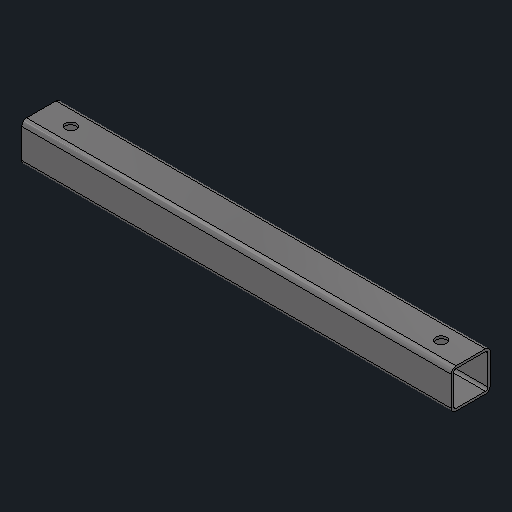
# Autodesk Inventor part: Model-4_Base Tube-1
Saved by Autodesk Inventor 2025.1 (Build 291241000, 241)
## iProperties
RuleStatus: InUse
Created: 2026-02-13
Part Number: Model-4_Base Tube-1
User Status: Released
Material: SS304
Description: Model-1 Base Tube-1
Document SubType Name: Modeling
Designer: Desktop -24
Density: 7.99949 g/cm^3
Appearance: Semi-Polished(1)
Mass: 20583.6 g
Surface Area: 8150.6 cm^2
Volume: 2573.11 cm^3
AfterDocNew0: Mat. Selection
encoded128: ÌStandard Î
encoded39: *STANDARD*
Family: SS304
Author: Desktop -24
Revision Number: 0
Autodesk Inventor part; units mm, degrees
ref_plane "YZ Plane" through (0, 0, 0) normal (1, 0, 0) x (0, 1, 0)
ref_plane "XZ Plane" through (0, 0, 0) normal (0, 1, 0) x (-1, 0, 0)
ref_plane "XY Plane" through (0, 0, 0) normal (0, 0, 1) x (1, 0, 0)
sketch "Sketch5" plane through (0, 0, 0) normal (1, 0, 0) x (0, 1, 0)
  line L0 (-38.1, 50.8) -> (38.1, 50.8)
  line L1 (50.8, 38.1) -> (50.8, -38.1)
  line L2 (38.1, -50.8) -> (-38.1, -50.8)
  line L3 (-50.8, -38.1) -> (-50.8, 38.1)
  line L4 (-50.8, 50.8) -> (50.8, -50.8) construction
  line L5 (50.8, 50.8) -> (-50.8, -50.8) construction
  arc A0 (50.8, 38.1) -> (38.1, 50.8) centre (38.1, 38.1) ccw
  arc A1 (38.1, -50.8) -> (50.8, -38.1) centre (38.1, -38.1) ccw
  arc A2 (-50.8, -38.1) -> (-38.1, -50.8) centre (-38.1, -38.1) ccw
  arc A3 (-38.1, 50.8) -> (-50.8, 38.1) centre (-38.1, 38.1) ccw
  line L6 (44.45, -38.1) -> (44.45, 38.1)
  arc A4 (44.45, 38.1) -> (38.1, 44.45) centre (38.1, 38.1) ccw
  line L7 (38.1, 44.45) -> (-38.1, 44.45)
  arc A5 (-38.1, 44.45) -> (-44.45, 38.1) centre (-38.1, 38.1) ccw
  line L8 (-44.45, 38.1) -> (-44.45, -38.1)
  arc A6 (-44.45, -38.1) -> (-38.1, -44.45) centre (-38.1, -38.1) ccw
  line L9 (-38.1, -44.45) -> (38.1, -44.45)
  arc A7 (38.1, -44.45) -> (44.45, -38.1) centre (38.1, -38.1) ccw
  point P0 (0, 0)
  dimension "d6" = 101.6
  dimension "d7" = 101.6
  dimension "d8" = 12.7
  dimension "d9" = 6.35
  constraints: 20 end point, 16 point on circle, 8 centre point, 8 point on line, 8 tangent, 4 parallel, 3 equal radius, 2 midpoint, 2 perpendicular, 1 horizontal, 7 other
  measures "d6" distance of L5.start L4.end
  measures "d7" distance of L4.end L5.end
  measures "d8" radius of A0
  measures "d9" distance between parallel lines of L1 L6
extrude "Extrusion4" add sketch "Sketch5" along normal mid plane 1111.25
sketch "Sketch9" plane through (-555.625, 50.8, 38.1) normal (0, 1, 0) x (1, 0, 0)
  line L0 (0, 38.1) -> (1111.25, 38.1) construction
  line L1 (1111.25, 0) -> (1111.25, 76.2) projected
  circle A0 centre (76.2, 38.1) radius 14.2875
  line L2 (0, 0) -> (0, 76.2) projected
  circle A1 centre (1035.05, 38.1) radius 14.2875
  point P0 (555.625, 38.1)
  dimension "d30" = 28.575
  dimension "d31" = 76.2
  dimension "d32" = 76.2
  constraints: 2 centre point, 2 end point, 2 midpoint, 2 point on line, 1 equal radius, 1 horizontal
  measures "d30" diameter of A0
  measures "d31" distance from line of L2 A0.centre
  measures "d32" distance from line of L1 A1.centre
extrude "Extrusion8" cut sketch "Sketch9" against normal blind 382.5875
body "Solid4"
